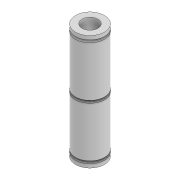
# Autodesk Inventor part: fullbar
Saved by Autodesk Inventor 2021 (Build 250183000, 183)
## iProperties
Created: 2022-10-12
Part Number: fullbar
Material: Generic
Document SubType Name: Modeling
Designer: alyn649
Density: 1 g/cm^3
Appearance: Default
Author: alyn649
Autodesk Inventor part; units mm, degrees
ref_plane "YZ Plane" through (0, 0, 0) normal (1, 0, 0) x (0, 1, 0)
sketch "Sketch1" plane through (0, 0, 0) normal (0, 1, 0) x (-1, 0, 0)
  circle A0 centre (0, 0) radius 2.9
  circle A1 centre (0, 0) radius 1.6
  dimension "d0" = 3.2
  dimension "d1" = 5.8
  constraints: 2 centre point, 2 coincident
  measures "d0" diameter of A1
  measures "d1" diameter of A0
extrude "Extrusion1" add sketch "Sketch1" along normal blind 23
ref_plane "Work Plane1" through (0, 11.5, 0) normal (0, 1, 0) x (1, 0, 0)
sketch "Sketch3" plane through (0, 11.5, 0) normal (0, 1, 0) x (1, 0, 0)
  circle A0 centre (0, 0) radius 1.6 construction
  circle A1 centre (0, 0) radius 2.2
  circle A2 centre (0, 0) radius 2.9 projected
  dimension "d12" = 0.7
  constraints: 1 centre point, 1 coincident
  measures "d12" radial gap between concentric circles of A2 A1
extrude "Extrusion3" cut sketch "Sketch3" along normal mid plane 0.5
ref_plane "Work Plane2" through (0, 22, 0) normal (0, 1, 0) x (1, 0, 0)
sketch "Sketch4" plane through (0, 22, 0) normal (0, 1, 0) x (1, 0, 0)
  circle A0 centre (0, 0) radius 2.9 projected
  circle A1 centre (0, 0) radius 2.2
  dimension "d9" = 0.7
  constraints: 1 centre point, 1 coincident
  measures "d9" radial gap between concentric circles of A0 A1
extrude "Extrusion4" cut sketch "Sketch4" along normal mid plane 0.5
mirror "Mirror1" about plane through (0, 11.5, 0) normal (0, 1, 0) of "Extrusion4"
body "Solid1"
